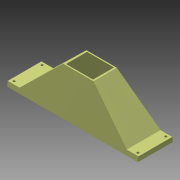
# Autodesk Inventor part: 集肉斗
Saved by Autodesk Inventor 2015 (Build 190159000, 159)
## iProperties
Created: 2017-05-22
Part Number: 集肉斗
Material: 常规
Document SubType Name: Modeling
Designer: Administrator
Density: 1 g/cm^3
Appearance: 缎光 - 柠檬绸色
Author: Administrator
Autodesk Inventor part; units mm, degrees
ref_plane "YZ Plane" through (0, 0, 0) normal (1, 0, 0) x (0, 1, 0)
ref_plane "XZ Plane" through (0, 0, 0) normal (0, 1, 0) x (-1, 0, 0)
sketch "草图1" plane through (0, 0, 0) normal (0, 0, 1) x (1, 0, 0)
  line L0 (-250, 75) -> (250, 75)
  line L1 (250, 75) -> (250, -75)
  line L2 (250, -75) -> (-250, -75)
  line L3 (-250, -75) -> (-250, 75)
  line L4 (0, 0) -> (2.8313, 0)
  line L5 (0, 0) -> (0, -2.8313)
  point P0 (0, 75)
  point P1 (250, 0)
  dimension "d0" = 2.8313
  dimension "d1" = 500
  dimension "d2" = 150
  constraints: 12 end point, 2 horizontal, 2 midpoint, 2 parallel, 2 perpendicular, 2 point on line, 1 vertical
  measures "d0" distance of L4.start L5.end
  measures "d1" distance of L0.start L0.end
  measures "d2" distance of L0.end L1.end
ref_plane "工作平面1" through (0, 0, 180) normal (0, 0, 1) x (1, 0, 0)
sketch "草图2" plane through (0, 0, 180) normal (0, 0, 1) x (1, 0, 0)
  line L0 (-65, 50) -> (65, 50)
  line L1 (65, 50) -> (65, -50)
  line L2 (65, -50) -> (-65, -50)
  line L3 (-65, -50) -> (-65, 50)
  line L4 (0, 0) -> (3.7262, 0)
  line L5 (0, 0) -> (0, -4.1463)
  point P0 (0, 50)
  point P1 (-65, 0)
  dimension "d4" = 130
  dimension "d5" = 100
  constraints: 12 end point, 2 horizontal, 2 midpoint, 2 parallel, 2 point on line, 1 perpendicular, 1 vertical
  measures "d4" distance of L0.start L0.end
  measures "d5" distance of L0.end L1.end
loft "放样1" add profiles "草图1", "草图2"
shell "抽壳1" thickness 5 removed faces 2 at (-83.3333, -25, 0) at (-21.6667, -16.6667, 180)
sketch "草图3" plane through (250, 75, 0) normal (0, 0, -1) x (-1, 0, 0)
  line L0 (530, 0) -> (-30, 0)
  line L1 (-30, 0) -> (-30, -150)
  line L2 (-30, -150) -> (530, -150)
  line L3 (530, -150) -> (530, 0)
  line L4 (500, 0) -> (0, 0) projected
  line L5 (0, -150) -> (500, -150) projected
  line L6 (0, 0) -> (0, -150) projected
  line L7 (500, -150) -> (500, 0) projected
  line L8 (492.8301, 0) -> (492.8301, -150)
  line L9 (7.1699, 0) -> (7.1699, -150)
  line L10 (0, -150) -> (185, -125) projected
  line L11 (492.8301, -5.048) -> (492.8301, -144.952) projected
  line L12 (7.1699, -144.952) -> (7.1699, -5.048) projected
  point P0 (250, -75)
  dimension "d11" = 30
  dimension "d12" = 30
  constraints: 12 end point, 4 collinear, 4 point on line, 3 parallel, 2 perpendicular, 1 horizontal
  measures "d11" distance between parallel lines of L1 L6
  measures "d12" distance between parallel lines of L7 L3
extrude "拉伸1" add sketch "草图3" against normal blind 20 contours L3 L2 L7 L0 | L7 L2 L8 L0 | L9 L10 L6 L0 | L6 L2 L1 L0 | L2 L10 L9
sketch "草图4" plane through (242.8301, 75, 0) normal (0, 1, 0) x (1, 0, 0)
  line L0 (0, -20) -> (-13.3856, -20)
  line L1 (-13.3856, -20) -> (0, -6.9762)
  line L2 (0, -6.9762) -> (-177.8301, -180) projected
  line L3 (0, -6.9762) -> (0, -20)
  line L4 (0, 0) -> (0, -20) projected
  line L5 (-485.6601, -20) -> (-472.2745, -20)
  line L6 (-472.2745, -20) -> (-485.6601, -6.9762)
  line L7 (-485.6601, -6.9762) -> (-307.8301, -180) projected
  line L8 (-485.6601, -6.9762) -> (-485.6601, -20)
  line L9 (-485.6601, 0) -> (-485.6601, -20) projected
  point P0 (-242.8301, 0)
  constraints: 12 end point, 4 collinear, 1 horizontal, 1 point on line
extrude "拉伸2" add sketch "草图4" against normal blind 150
sketch "草图5" plane through (280, -75, 0) normal (1, 0, 0) x (0, 0, -1)
  line L0 (0, 150) -> (-20, 147.2222)
  line L1 (-6.9762, 149.0311) -> (-20, 147.2222) projected
  line L2 (-20, 147.2222) -> (-20, 150)
  line L3 (-20, 150) -> (0, 150)
  line L4 (-20, 147.2222) -> (-180, 125) projected
  line L5 (0, 0) -> (-20, 0)
  line L6 (0, 0) -> (-20, 0) projected
  line L7 (-20, 0) -> (-20, 2.8101)
  line L8 (-20, 150) -> (-20, 0) projected
  line L9 (0, 0) -> (-20, 2.7778)
  line L10 (-6.9762, 0.9689) -> (-20, 2.7778) projected
  point P0 (0, 75)
  constraints: 12 end point, 4 collinear, 1 perpendicular, 1 point on line
extrude "拉伸3" cut sketch "草图5" against normal through all
sketch "草图6" plane through (280, -75, 0) normal (0, 0, -1) x (-1, 0, 0)
  circle A0 centre (545, 135) radius 12.5
  circle A1 centre (545, 15) radius 12.5
  circle A2 centre (15, 135) radius 12.5
  circle A3 centre (15, 15) radius 12.5
  line L0 (560, 150) -> (0, 150) projected
  line L1 (560, 0) -> (560, 150) projected
  line L2 (0, 0) -> (560, 0) projected
  line L3 (0, 150) -> (0, 0) projected
  point P0 (280, 75)
  dimension "d19" = 25
  dimension "d20" = 25
  dimension "d21" = 25
  dimension "d22" = 25
  dimension "d23" = 15
  dimension "d24" = 15
  dimension "d25" = 15
  dimension "d26" = 15
  dimension "d27" = 15
  dimension "d28" = 15
  dimension "d29" = 15
  dimension "d30" = 15
  constraints: 4 centre point
  measures "d19" diameter of A0
  measures "d20" diameter of A1
  measures "d21" diameter of A2
  measures "d22" diameter of A3
  measures "d23" distance from line of L0 A0.centre
  measures "d24" distance from line of L1 A0.centre
  measures "d25" distance from line of L2 A1.centre
  measures "d26" distance from line of L1 A1.centre
  measures "d27" distance from line of A3.centre L2
  measures "d28" distance from line of L3 A3.centre
  measures "d29" distance from line of L3 A2.centre
  measures "d30" distance from line of L0 A2.centre
extrude "拉伸4" cut sketch "草图6" against normal blind 10 contours A0 | A1 | A2 | A3
sketch "草图7" plane through (-265, 60, 10) normal (0, 0, -1) x (-1, 0, 0)
  circle A0 centre (0, 0) radius 5
  circle A1 centre (0, -120) radius 5
  circle A2 centre (-530, -120) radius 5
  circle A3 centre (-530, 0) radius 5
  circle A4 centre (0, 0) radius 12.5 projected
  circle A5 centre (0, -120) radius 12.5 projected
  circle A6 centre (-530, -120) radius 12.5 projected
  circle A7 centre (-530, 0) radius 12.5 projected
  point P0 (-265, -60)
  dimension "d33" = 10
  dimension "d34" = 10
  dimension "d35" = 10
  dimension "d36" = 10
  constraints: 4 centre point, 4 concentric
  measures "d33" diameter of A0
  measures "d34" diameter of A1
  measures "d35" diameter of A2
  measures "d36" diameter of A3
extrude "拉伸5" cut sketch "草图7" against normal blind 10 contours A0 | A1 | A2 | A3
